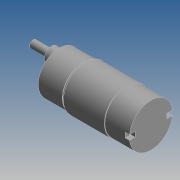
# Autodesk Inventor part: Moteur
Saved by Autodesk Inventor 2012 SP1 (Build 160190100, 190)
## iProperties
Created: 2012-07-09
Part Number: Moteur
Material: Default
Document SubType Name: Modeling
Designer: sta
Density: 1 g/cm^3
Author: sta
Autodesk Inventor part; units mm, degrees
ref_plane "YZ Plane" through (0, 0, 0) normal (1, 0, 0) x (0, 1, 0)
ref_plane "XZ Plane" through (0, 0, 0) normal (0, 1, 0) x (-1, 0, 0)
ref_plane "XY Plane" through (0, 0, 0) normal (0, 0, 1) x (1, 0, 0)
sketch "Sketch1" plane through (0, 0, 0) normal (0, 0, 1) x (1, 0, 0)
  line L0 (0, 0) -> (76.5, 0)
  line L1 (0, 0) -> (0, 17.5)
  line L2 (0, 17.5) -> (20, 17.5)
  line L3 (20, 17.5) -> (20, 17)
  line L4 (20, 17) -> (22, 17)
  line L5 (22, 17) -> (22, 18.5)
  line L6 (22, 18.5) -> (56.1, 18.5)
  line L7 (56.1, 18.5) -> (56.1, 18)
  line L8 (56.1, 18) -> (76.5, 18)
  line L9 (76.5, 18) -> (76.5, 0)
  dimension "d0" = 76.5
  dimension "d1" = 34
  dimension "d2" = 35
  dimension "d3" = 37
  dimension "d4" = 36
  dimension "d5" = 20
  dimension "d6" = 2
  dimension "d7" = 34.1
  constraints: 20 end point, 7 parallel, 2 perpendicular, 1 horizontal
  measures "d0" distance of L0.start L0.end
  measures "d1" diameter of L4 L0
  measures "d2" diameter of L2 L0
  measures "d3" diameter of L6 L0
  measures "d4" diameter of L8 L0
  measures "d5" distance from line of L2.end L1
  measures "d6" distance of L3.end L4.end
  measures "d7" distance of L5.end L6.end
revolve "Revolution1" add sketch "Sketch1" angle 360 about axis through (0, 0, 0) along (1, 0, 0)
sketch "Sketch2" plane through (76.5, 0, 0) normal (1, 0, 0) x (0, 0, -1)
  line L0 (-2.05, 20.1398) -> (2.05, 20.1398)
  line L1 (2.05, 20.1398) -> (2.05, 13.25)
  line L2 (2.05, 13.25) -> (-2.05, 13.25)
  line L3 (-2.05, 13.25) -> (-2.05, 20.1398)
  line L4 (-2.05, -13.25) -> (2.05, -13.25)
  line L5 (2.05, -13.25) -> (2.05, -20.9754)
  line L6 (2.05, -20.9754) -> (-2.05, -20.9754)
  line L7 (-2.05, -20.9754) -> (-2.05, -13.25)
  point P0 (0, 0)
  dimension "d9" = 4.1
  dimension "d10" = 4.1
  dimension "d11" = 2.05
  dimension "d12" = 2.05
  dimension "d13" = 26.5
  dimension "d14" = 13.25
  constraints: 16 end point, 4 parallel, 2 horizontal, 2 perpendicular
  measures "d9" distance of L0.start L0.end
  measures "d10" distance of L5.end L6.end
  measures "d11" distance from line of L7 point (0, 0)
  measures "d12" distance from line of L3 point (0, 0)
  measures "d13" distance between parallel lines of L4 L2
  measures "d14" distance from line of point (0, 0) L2
extrude "Extrusion1" cut sketch "Sketch2" against normal blind 3.6
sketch "Sketch3" plane through (0, 0, 0) normal (-1, 0, 0) x (0, 0, 1)
  circle A0 centre (0, 0) radius 15.425 construction
  circle A1 centre (0, 15.425) radius 1.18
  dimension "d17" = 30.85
  dimension "d18" = 2.36
  constraints: 2 coincident, 1 centre point, 1 vertical alignment, 2 other
  measures "d18" diameter of A1
extrude "Extrusion2" add sketch "Sketch3" along normal blind 1.3
fillet "Fillet1" radius 1 1 edges at (-1.3, 15.425, -1.18)
pattern_circular "Circular Pattern1" count 3 over 360 about axis through (39.05, 0, 0) along (1, 0, 0) of "Extrusion2", "Fillet1"
sketch "Sketch4" plane through (0, 0, 0) normal (-1, 0, 0) x (0, 0, 1)
  circle A0 centre (0, 15.425) radius 1.18 construction
  circle A1 centre (13.3584, -7.7125) radius 1.18 construction
  line L0 (0, 15.425) -> (13.3584, -7.7125) construction
  line L1 (6.6792, 3.8563) -> (24.6731, 14.245) construction
  circle A2 centre (6.1661, 3.56) radius 6
  point P0 (0, 0)
  dimension "d25" = 7.12
  dimension "d26" = 12
  constraints: 4 end point, 1 centre point, 1 coincident, 1 midpoint, 1 perpendicular, 1 point on line
  measures "d25" distance of point (6.166, 3.56) point (0, 0)
  measures "d26" diameter of A2
extrude "Extrusion3" add sketch "Sketch4" along normal blind 10
sketch "Sketch5" plane through (-10, 3.56, 6.1661) normal (-1, 0, 0) x (0, 0, 1)
  circle A0 centre (0, 0) radius 6 construction
  circle A1 centre (0, 0) radius 3
  point P0 (-6.1661, -3.56)
  dimension "d29" = 6
  constraints: 1 centre point, 1 coincident
  measures "d29" diameter of A1
extrude "Extrusion4" add sketch "Sketch5" along normal blind 15.2
sketch "Sketch6" plane through (-25.2, 3.56, 6.1661) normal (-1, 0, 0) x (0, 0, 1)
  circle A0 centre (0, 0) radius 3 construction
  arc A1 (1.6583, 2.5) -> (-1.6583, 2.5) centre (0, 0) ccw
  line L0 (-1.6583, 2.5) -> (1.6583, 2.5)
  point P0 (-6.1661, -3.56)
  dimension "d35" = 2.5
  constraints: 4 point on circle, 2 end point, 1 centre point, 1 coincident, 1 horizontal
  measures "d35" distance from line of L0 A0.centre
extrude "Extrusion5" cut sketch "Sketch6" against normal blind 12
equation "\"d11\" = 0.5 * d10"
equation "\"d12\" = 0.5 * d9"
equation "\"d14\" = 0.5 * d13"
body "Solid1"
